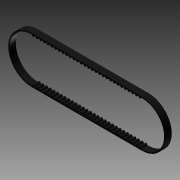
# Autodesk Inventor part: large drive belt
Saved by Autodesk Inventor 2012 (Build 160160000, 160)
## iProperties
Created: 2013-11-05
Part Number: large drive belt
Material: Default
Document SubType Name: Modeling
Designer: Bryce
Density: 1 g/cm^3
Author: Bryce
Autodesk Inventor part; units mm, degrees
ref_plane "YZ Plane" through (0, 0, 0) normal (1, 0, 0) x (0, 1, 0)
ref_plane "XZ Plane" through (0, 0, 0) normal (0, 1, 0) x (-1, 0, 0)
ref_plane "XY Plane" through (0, 0, 0) normal (0, 0, 1) x (1, 0, 0)
sketch "Sketch1" plane through (0, 0, 0) normal (0, 0, 1) x (1, 0, 0)
  arc A0 (0, 31.2674) -> (0, -31.2674) centre (0, 0) ccw
  arc A1 (155.575, -31.2674) -> (155.575, 31.2674) centre (155.575, 0) ccw
  line L0 (0, 31.2674) -> (155.575, 31.2674)
  line L1 (0, -31.2674) -> (4.3647, -31.2674)
  arc A2 (155.575, -33.02) -> (155.575, 33.02) centre (155.575, 0) ccw
  line L2 (155.575, -33.02) -> (0, -33.02)
  arc A3 (0, 33.02) -> (0, -33.02) centre (0, 0) ccw
  line L3 (0, 33.02) -> (155.575, 33.02)
  arc A4 (3.7592, -30.7283) -> (0.6055, -30.7283) centre (2.1824, -30.9118) ccw
  arc A5 (0, -31.2674) -> (0.6055, -30.7283) centre (0, -30.6578) ccw
  arc A6 (3.7592, -30.7283) -> (4.3647, -31.2674) centre (4.3647, -30.6578) ccw
  line L4 (4.3647, -31.2674) -> (155.575, -31.2674)
  line L5 (5.1816, -31.2674) -> (9.5463, -31.2674)
  arc A7 (8.9408, -30.7283) -> (5.7871, -30.7283) centre (7.364, -30.9118) ccw
  arc A8 (5.1816, -31.2674) -> (5.7871, -30.7283) centre (5.1816, -30.6578) ccw
  arc A9 (8.9408, -30.7283) -> (9.5463, -31.2674) centre (9.5463, -30.6578) ccw
  line L6 (10.3632, -31.2674) -> (14.7279, -31.2674)
  arc A10 (14.1224, -30.7283) -> (10.9687, -30.7283) centre (12.5456, -30.9118) ccw
  arc A11 (10.3632, -31.2674) -> (10.9687, -30.7283) centre (10.3632, -30.6578) ccw
  arc A12 (14.1224, -30.7283) -> (14.7279, -31.2674) centre (14.7279, -30.6578) ccw
  line L7 (15.5448, -31.2674) -> (19.9095, -31.2674)
  arc A13 (19.304, -30.7283) -> (16.1503, -30.7283) centre (17.7272, -30.9118) ccw
  arc A14 (15.5448, -31.2674) -> (16.1503, -30.7283) centre (15.5448, -30.6578) ccw
  arc A15 (19.304, -30.7283) -> (19.9095, -31.2674) centre (19.9095, -30.6578) ccw
  line L8 (20.7264, -31.2674) -> (25.0911, -31.2674)
  arc A16 (24.4856, -30.7283) -> (21.3319, -30.7283) centre (22.9088, -30.9118) ccw
  arc A17 (20.7264, -31.2674) -> (21.3319, -30.7283) centre (20.7264, -30.6578) ccw
  arc A18 (24.4856, -30.7283) -> (25.0911, -31.2674) centre (25.0911, -30.6578) ccw
  line L9 (25.908, -31.2674) -> (30.2727, -31.2674)
  arc A19 (29.6672, -30.7283) -> (26.5135, -30.7283) centre (28.0904, -30.9118) ccw
  arc A20 (25.908, -31.2674) -> (26.5135, -30.7283) centre (25.908, -30.6578) ccw
  arc A21 (29.6672, -30.7283) -> (30.2727, -31.2674) centre (30.2727, -30.6578) ccw
  line L10 (31.0896, -31.2674) -> (35.4543, -31.2674)
  arc A22 (34.8488, -30.7283) -> (31.6951, -30.7283) centre (33.272, -30.9118) ccw
  arc A23 (31.0896, -31.2674) -> (31.6951, -30.7283) centre (31.0896, -30.6578) ccw
  arc A24 (34.8488, -30.7283) -> (35.4543, -31.2674) centre (35.4543, -30.6578) ccw
  line L11 (36.2712, -31.2674) -> (40.6359, -31.2674)
  arc A25 (40.0304, -30.7283) -> (36.8767, -30.7283) centre (38.4536, -30.9118) ccw
  arc A26 (36.2712, -31.2674) -> (36.8767, -30.7283) centre (36.2712, -30.6578) ccw
  arc A27 (40.0304, -30.7283) -> (40.6359, -31.2674) centre (40.6359, -30.6578) ccw
  line L12 (41.4528, -31.2674) -> (45.8175, -31.2674)
  arc A28 (45.212, -30.7283) -> (42.0583, -30.7283) centre (43.6352, -30.9118) ccw
  arc A29 (41.4528, -31.2674) -> (42.0583, -30.7283) centre (41.4528, -30.6578) ccw
  arc A30 (45.212, -30.7283) -> (45.8175, -31.2674) centre (45.8175, -30.6578) ccw
  line L13 (46.6344, -31.2674) -> (50.9991, -31.2674)
  arc A31 (50.3936, -30.7283) -> (47.2399, -30.7283) centre (48.8168, -30.9118) ccw
  arc A32 (46.6344, -31.2674) -> (47.2399, -30.7283) centre (46.6344, -30.6578) ccw
  arc A33 (50.3936, -30.7283) -> (50.9991, -31.2674) centre (50.9991, -30.6578) ccw
  line L14 (51.816, -31.2674) -> (56.1807, -31.2674)
  arc A34 (55.5752, -30.7283) -> (52.4215, -30.7283) centre (53.9984, -30.9118) ccw
  arc A35 (51.816, -31.2674) -> (52.4215, -30.7283) centre (51.816, -30.6578) ccw
  arc A36 (55.5752, -30.7283) -> (56.1807, -31.2674) centre (56.1807, -30.6578) ccw
  line L15 (56.9976, -31.2674) -> (61.3623, -31.2674)
  arc A37 (60.7568, -30.7283) -> (57.6031, -30.7283) centre (59.18, -30.9118) ccw
  arc A38 (56.9976, -31.2674) -> (57.6031, -30.7283) centre (56.9976, -30.6578) ccw
  arc A39 (60.7568, -30.7283) -> (61.3623, -31.2674) centre (61.3623, -30.6578) ccw
  line L16 (62.1792, -31.2674) -> (66.5439, -31.2674)
  arc A40 (65.9384, -30.7283) -> (62.7847, -30.7283) centre (64.3616, -30.9118) ccw
  arc A41 (62.1792, -31.2674) -> (62.7847, -30.7283) centre (62.1792, -30.6578) ccw
  arc A42 (65.9384, -30.7283) -> (66.5439, -31.2674) centre (66.5439, -30.6578) ccw
  line L17 (67.3608, -31.2674) -> (71.7255, -31.2674)
  arc A43 (71.12, -30.7283) -> (67.9663, -30.7283) centre (69.5432, -30.9118) ccw
  arc A44 (67.3608, -31.2674) -> (67.9663, -30.7283) centre (67.3608, -30.6578) ccw
  arc A45 (71.12, -30.7283) -> (71.7255, -31.2674) centre (71.7255, -30.6578) ccw
  line L18 (72.5424, -31.2674) -> (76.9071, -31.2674)
  arc A46 (76.3016, -30.7283) -> (73.1479, -30.7283) centre (74.7248, -30.9118) ccw
  arc A47 (72.5424, -31.2674) -> (73.1479, -30.7283) centre (72.5424, -30.6578) ccw
  arc A48 (76.3016, -30.7283) -> (76.9071, -31.2674) centre (76.9071, -30.6578) ccw
  line L19 (77.724, -31.2674) -> (82.0887, -31.2674)
  arc A49 (81.4832, -30.7283) -> (78.3295, -30.7283) centre (79.9064, -30.9118) ccw
  arc A50 (77.724, -31.2674) -> (78.3295, -30.7283) centre (77.724, -30.6578) ccw
  arc A51 (81.4832, -30.7283) -> (82.0887, -31.2674) centre (82.0887, -30.6578) ccw
  line L20 (82.9056, -31.2674) -> (87.2703, -31.2674)
  arc A52 (86.6648, -30.7283) -> (83.5111, -30.7283) centre (85.088, -30.9118) ccw
  arc A53 (82.9056, -31.2674) -> (83.5111, -30.7283) centre (82.9056, -30.6578) ccw
  arc A54 (86.6648, -30.7283) -> (87.2703, -31.2674) centre (87.2703, -30.6578) ccw
  line L21 (88.0872, -31.2674) -> (92.4519, -31.2674)
  arc A55 (91.8464, -30.7283) -> (88.6927, -30.7283) centre (90.2696, -30.9118) ccw
  arc A56 (88.0872, -31.2674) -> (88.6927, -30.7283) centre (88.0872, -30.6578) ccw
  arc A57 (91.8464, -30.7283) -> (92.4519, -31.2674) centre (92.4519, -30.6578) ccw
  line L22 (93.2688, -31.2674) -> (97.6335, -31.2674)
  arc A58 (97.028, -30.7283) -> (93.8743, -30.7283) centre (95.4512, -30.9118) ccw
  arc A59 (93.2688, -31.2674) -> (93.8743, -30.7283) centre (93.2688, -30.6578) ccw
  arc A60 (97.028, -30.7283) -> (97.6335, -31.2674) centre (97.6335, -30.6578) ccw
  line L23 (98.4504, -31.2674) -> (102.8151, -31.2674)
  arc A61 (102.2096, -30.7283) -> (99.0559, -30.7283) centre (100.6328, -30.9118) ccw
  arc A62 (98.4504, -31.2674) -> (99.0559, -30.7283) centre (98.4504, -30.6578) ccw
  arc A63 (102.2096, -30.7283) -> (102.8151, -31.2674) centre (102.8151, -30.6578) ccw
  line L24 (103.632, -31.2674) -> (107.9967, -31.2674)
  arc A64 (107.3912, -30.7283) -> (104.2375, -30.7283) centre (105.8144, -30.9118) ccw
  arc A65 (103.632, -31.2674) -> (104.2375, -30.7283) centre (103.632, -30.6578) ccw
  arc A66 (107.3912, -30.7283) -> (107.9967, -31.2674) centre (107.9967, -30.6578) ccw
  line L25 (108.8136, -31.2674) -> (113.1783, -31.2674)
  arc A67 (112.5728, -30.7283) -> (109.4191, -30.7283) centre (110.996, -30.9118) ccw
  arc A68 (108.8136, -31.2674) -> (109.4191, -30.7283) centre (108.8136, -30.6578) ccw
  arc A69 (112.5728, -30.7283) -> (113.1783, -31.2674) centre (113.1783, -30.6578) ccw
  line L26 (113.9952, -31.2674) -> (118.3599, -31.2674)
  arc A70 (117.7544, -30.7283) -> (114.6007, -30.7283) centre (116.1776, -30.9118) ccw
  arc A71 (113.9952, -31.2674) -> (114.6007, -30.7283) centre (113.9952, -30.6578) ccw
  arc A72 (117.7544, -30.7283) -> (118.3599, -31.2674) centre (118.3599, -30.6578) ccw
  line L27 (119.1768, -31.2674) -> (123.5415, -31.2674)
  arc A73 (122.936, -30.7283) -> (119.7823, -30.7283) centre (121.3592, -30.9118) ccw
  arc A74 (119.1768, -31.2674) -> (119.7823, -30.7283) centre (119.1768, -30.6578) ccw
  arc A75 (122.936, -30.7283) -> (123.5415, -31.2674) centre (123.5415, -30.6578) ccw
  line L28 (124.3584, -31.2674) -> (128.7231, -31.2674)
  arc A76 (128.1176, -30.7283) -> (124.9639, -30.7283) centre (126.5408, -30.9118) ccw
  arc A77 (124.3584, -31.2674) -> (124.9639, -30.7283) centre (124.3584, -30.6578) ccw
  arc A78 (128.1176, -30.7283) -> (128.7231, -31.2674) centre (128.7231, -30.6578) ccw
  line L29 (129.54, -31.2674) -> (133.9047, -31.2674)
  arc A79 (133.2992, -30.7283) -> (130.1455, -30.7283) centre (131.7224, -30.9118) ccw
  arc A80 (129.54, -31.2674) -> (130.1455, -30.7283) centre (129.54, -30.6578) ccw
  arc A81 (133.2992, -30.7283) -> (133.9047, -31.2674) centre (133.9047, -30.6578) ccw
  line L30 (134.7216, -31.2674) -> (139.0863, -31.2674)
  arc A82 (138.4808, -30.7283) -> (135.3271, -30.7283) centre (136.904, -30.9118) ccw
  arc A83 (134.7216, -31.2674) -> (135.3271, -30.7283) centre (134.7216, -30.6578) ccw
  arc A84 (138.4808, -30.7283) -> (139.0863, -31.2674) centre (139.0863, -30.6578) ccw
  line L31 (139.9032, -31.2674) -> (144.2679, -31.2674)
  arc A85 (143.6624, -30.7283) -> (140.5087, -30.7283) centre (142.0856, -30.9118) ccw
  arc A86 (139.9032, -31.2674) -> (140.5087, -30.7283) centre (139.9032, -30.6578) ccw
  arc A87 (143.6624, -30.7283) -> (144.2679, -31.2674) centre (144.2679, -30.6578) ccw
  line L32 (145.0848, -31.2674) -> (149.4495, -31.2674)
  arc A88 (148.844, -30.7283) -> (145.6903, -30.7283) centre (147.2672, -30.9118) ccw
  arc A89 (145.0848, -31.2674) -> (145.6903, -30.7283) centre (145.0848, -30.6578) ccw
  arc A90 (148.844, -30.7283) -> (149.4495, -31.2674) centre (149.4495, -30.6578) ccw
  line L33 (150.2664, -31.2674) -> (154.6311, -31.2674)
  arc A91 (154.0256, -30.7283) -> (150.8719, -30.7283) centre (152.4488, -30.9118) ccw
  arc A92 (150.2664, -31.2674) -> (150.8719, -30.7283) centre (150.2664, -30.6578) ccw
  arc A93 (154.0256, -30.7283) -> (154.6311, -31.2674) centre (154.6311, -30.6578) ccw
  line L34 (0, 0) -> (155.575, 0) construction
  line L35 (0, 31.2674) -> (4.3647, 31.2674)
  arc A94 (0.6055, 30.7283) -> (3.7592, 30.7283) centre (2.1824, 30.9118) ccw
  arc A95 (0.6055, 30.7283) -> (0, 31.2674) centre (0, 30.6578) ccw
  arc A96 (4.3647, 31.2674) -> (3.7592, 30.7283) centre (4.3647, 30.6578) ccw
  line L36 (5.1816, 31.2674) -> (9.5463, 31.2674)
  arc A97 (5.7871, 30.7283) -> (8.9408, 30.7283) centre (7.364, 30.9118) ccw
  arc A98 (5.7871, 30.7283) -> (5.1816, 31.2674) centre (5.1816, 30.6578) ccw
  arc A99 (9.5463, 31.2674) -> (8.9408, 30.7283) centre (9.5463, 30.6578) ccw
  line L37 (10.3632, 31.2674) -> (14.7279, 31.2674)
  arc A100 (10.9687, 30.7283) -> (14.1224, 30.7283) centre (12.5456, 30.9118) ccw
  arc A101 (10.9687, 30.7283) -> (10.3632, 31.2674) centre (10.3632, 30.6578) ccw
  arc A102 (14.7279, 31.2674) -> (14.1224, 30.7283) centre (14.7279, 30.6578) ccw
  line L38 (15.5448, 31.2674) -> (19.9095, 31.2674)
  arc A103 (16.1503, 30.7283) -> (19.304, 30.7283) centre (17.7272, 30.9118) ccw
  arc A104 (16.1503, 30.7283) -> (15.5448, 31.2674) centre (15.5448, 30.6578) ccw
  arc A105 (19.9095, 31.2674) -> (19.304, 30.7283) centre (19.9095, 30.6578) ccw
  line L39 (20.7264, 31.2674) -> (25.0911, 31.2674)
  arc A106 (21.3319, 30.7283) -> (24.4856, 30.7283) centre (22.9088, 30.9118) ccw
  arc A107 (21.3319, 30.7283) -> (20.7264, 31.2674) centre (20.7264, 30.6578) ccw
  arc A108 (25.0911, 31.2674) -> (24.4856, 30.7283) centre (25.0911, 30.6578) ccw
  line L40 (25.908, 31.2674) -> (30.2727, 31.2674)
  arc A109 (26.5135, 30.7283) -> (29.6672, 30.7283) centre (28.0904, 30.9118) ccw
  arc A110 (26.5135, 30.7283) -> (25.908, 31.2674) centre (25.908, 30.6578) ccw
  arc A111 (30.2727, 31.2674) -> (29.6672, 30.7283) centre (30.2727, 30.6578) ccw
  line L41 (31.0896, 31.2674) -> (35.4543, 31.2674)
  arc A112 (31.6951, 30.7283) -> (34.8488, 30.7283) centre (33.272, 30.9118) ccw
  arc A113 (31.6951, 30.7283) -> (31.0896, 31.2674) centre (31.0896, 30.6578) ccw
  arc A114 (35.4543, 31.2674) -> (34.8488, 30.7283) centre (35.4543, 30.6578) ccw
  line L42 (36.2712, 31.2674) -> (40.6359, 31.2674)
  arc A115 (36.8767, 30.7283) -> (40.0304, 30.7283) centre (38.4536, 30.9118) ccw
  arc A116 (36.8767, 30.7283) -> (36.2712, 31.2674) centre (36.2712, 30.6578) ccw
  arc A117 (40.6359, 31.2674) -> (40.0304, 30.7283) centre (40.6359, 30.6578) ccw
  line L43 (41.4528, 31.2674) -> (45.8175, 31.2674)
  arc A118 (42.0583, 30.7283) -> (45.212, 30.7283) centre (43.6352, 30.9118) ccw
  arc A119 (42.0583, 30.7283) -> (41.4528, 31.2674) centre (41.4528, 30.6578) ccw
  arc A120 (45.8175, 31.2674) -> (45.212, 30.7283) centre (45.8175, 30.6578) ccw
  line L44 (46.6344, 31.2674) -> (50.9991, 31.2674)
  arc A121 (47.2399, 30.7283) -> (50.3936, 30.7283) centre (48.8168, 30.9118) ccw
  arc A122 (47.2399, 30.7283) -> (46.6344, 31.2674) centre (46.6344, 30.6578) ccw
  arc A123 (50.9991, 31.2674) -> (50.3936, 30.7283) centre (50.9991, 30.6578) ccw
  line L45 (51.816, 31.2674) -> (56.1807, 31.2674)
  arc A124 (52.4215, 30.7283) -> (55.5752, 30.7283) centre (53.9984, 30.9118) ccw
  arc A125 (52.4215, 30.7283) -> (51.816, 31.2674) centre (51.816, 30.6578) ccw
  arc A126 (56.1807, 31.2674) -> (55.5752, 30.7283) centre (56.1807, 30.6578) ccw
  line L46 (56.9976, 31.2674) -> (61.3623, 31.2674)
  arc A127 (57.6031, 30.7283) -> (60.7568, 30.7283) centre (59.18, 30.9118) ccw
  arc A128 (57.6031, 30.7283) -> (56.9976, 31.2674) centre (56.9976, 30.6578) ccw
  arc A129 (61.3623, 31.2674) -> (60.7568, 30.7283) centre (61.3623, 30.6578) ccw
  line L47 (62.1792, 31.2674) -> (66.5439, 31.2674)
  arc A130 (62.7847, 30.7283) -> (65.9384, 30.7283) centre (64.3616, 30.9118) ccw
  arc A131 (62.7847, 30.7283) -> (62.1792, 31.2674) centre (62.1792, 30.6578) ccw
  arc A132 (66.5439, 31.2674) -> (65.9384, 30.7283) centre (66.5439, 30.6578) ccw
  line L48 (67.3608, 31.2674) -> (71.7255, 31.2674)
  arc A133 (67.9663, 30.7283) -> (71.12, 30.7283) centre (69.5432, 30.9118) ccw
  arc A134 (67.9663, 30.7283) -> (67.3608, 31.2674) centre (67.3608, 30.6578) ccw
  arc A135 (71.7255, 31.2674) -> (71.12, 30.7283) centre (71.7255, 30.6578) ccw
  line L49 (72.5424, 31.2674) -> (76.9071, 31.2674)
  arc A136 (73.1479, 30.7283) -> (76.3016, 30.7283) centre (74.7248, 30.9118) ccw
  arc A137 (73.1479, 30.7283) -> (72.5424, 31.2674) centre (72.5424, 30.6578) ccw
  arc A138 (76.9071, 31.2674) -> (76.3016, 30.7283) centre (76.9071, 30.6578) ccw
  line L50 (77.724, 31.2674) -> (82.0887, 31.2674)
  arc A139 (78.3295, 30.7283) -> (81.4832, 30.7283) centre (79.9064, 30.9118) ccw
  arc A140 (78.3295, 30.7283) -> (77.724, 31.2674) centre (77.724, 30.6578) ccw
  arc A141 (82.0887, 31.2674) -> (81.4832, 30.7283) centre (82.0887, 30.6578) ccw
  line L51 (82.9056, 31.2674) -> (87.2703, 31.2674)
  arc A142 (83.5111, 30.7283) -> (86.6648, 30.7283) centre (85.088, 30.9118) ccw
  arc A143 (83.5111, 30.7283) -> (82.9056, 31.2674) centre (82.9056, 30.6578) ccw
  arc A144 (87.2703, 31.2674) -> (86.6648, 30.7283) centre (87.2703, 30.6578) ccw
  line L52 (88.0872, 31.2674) -> (92.4519, 31.2674)
  arc A145 (88.6927, 30.7283) -> (91.8464, 30.7283) centre (90.2696, 30.9118) ccw
  arc A146 (88.6927, 30.7283) -> (88.0872, 31.2674) centre (88.0872, 30.6578) ccw
  arc A147 (92.4519, 31.2674) -> (91.8464, 30.7283) centre (92.4519, 30.6578) ccw
  line L53 (93.2688, 31.2674) -> (97.6335, 31.2674)
  arc A148 (93.8743, 30.7283) -> (97.028, 30.7283) centre (95.4512, 30.9118) ccw
  arc A149 (93.8743, 30.7283) -> (93.2688, 31.2674) centre (93.2688, 30.6578) ccw
  arc A150 (97.6335, 31.2674) -> (97.028, 30.7283) centre (97.6335, 30.6578) ccw
  line L54 (98.4504, 31.2674) -> (102.8151, 31.2674)
  arc A151 (99.0559, 30.7283) -> (102.2096, 30.7283) centre (100.6328, 30.9118) ccw
  arc A152 (99.0559, 30.7283) -> (98.4504, 31.2674) centre (98.4504, 30.6578) ccw
  arc A153 (102.8151, 31.2674) -> (102.2096, 30.7283) centre (102.8151, 30.6578) ccw
  line L55 (103.632, 31.2674) -> (107.9967, 31.2674)
  arc A154 (104.2375, 30.7283) -> (107.3912, 30.7283) centre (105.8144, 30.9118) ccw
  arc A155 (104.2375, 30.7283) -> (103.632, 31.2674) centre (103.632, 30.6578) ccw
  arc A156 (107.9967, 31.2674) -> (107.3912, 30.7283) centre (107.9967, 30.6578) ccw
  line L56 (108.8136, 31.2674) -> (113.1783, 31.2674)
  arc A157 (109.4191, 30.7283) -> (112.5728, 30.7283) centre (110.996, 30.9118) ccw
  arc A158 (109.4191, 30.7283) -> (108.8136, 31.2674) centre (108.8136, 30.6578) ccw
  arc A159 (113.1783, 31.2674) -> (112.5728, 30.7283) centre (113.1783, 30.6578) ccw
  line L57 (113.9952, 31.2674) -> (118.3599, 31.2674)
  arc A160 (114.6007, 30.7283) -> (117.7544, 30.7283) centre (116.1776, 30.9118) ccw
  arc A161 (114.6007, 30.7283) -> (113.9952, 31.2674) centre (113.9952, 30.6578) ccw
  arc A162 (118.3599, 31.2674) -> (117.7544, 30.7283) centre (118.3599, 30.6578) ccw
  line L58 (119.1768, 31.2674) -> (123.5415, 31.2674)
  arc A163 (119.7823, 30.7283) -> (122.936, 30.7283) centre (121.3592, 30.9118) ccw
  arc A164 (119.7823, 30.7283) -> (119.1768, 31.2674) centre (119.1768, 30.6578) ccw
  arc A165 (123.5415, 31.2674) -> (122.936, 30.7283) centre (123.5415, 30.6578) ccw
  line L59 (124.3584, 31.2674) -> (128.7231, 31.2674)
  arc A166 (124.9639, 30.7283) -> (128.1176, 30.7283) centre (126.5408, 30.9118) ccw
  arc A167 (124.9639, 30.7283) -> (124.3584, 31.2674) centre (124.3584, 30.6578) ccw
  arc A168 (128.7231, 31.2674) -> (128.1176, 30.7283) centre (128.7231, 30.6578) ccw
  line L60 (129.54, 31.2674) -> (133.9047, 31.2674)
  arc A169 (130.1455, 30.7283) -> (133.2992, 30.7283) centre (131.7224, 30.9118) ccw
  arc A170 (130.1455, 30.7283) -> (129.54, 31.2674) centre (129.54, 30.6578) ccw
  arc A171 (133.9047, 31.2674) -> (133.2992, 30.7283) centre (133.9047, 30.6578) ccw
  line L61 (134.7216, 31.2674) -> (139.0863, 31.2674)
  arc A172 (135.3271, 30.7283) -> (138.4808, 30.7283) centre (136.904, 30.9118) ccw
  arc A173 (135.3271, 30.7283) -> (134.7216, 31.2674) centre (134.7216, 30.6578) ccw
  arc A174 (139.0863, 31.2674) -> (138.4808, 30.7283) centre (139.0863, 30.6578) ccw
  line L62 (139.9032, 31.2674) -> (144.2679, 31.2674)
  arc A175 (140.5087, 30.7283) -> (143.6624, 30.7283) centre (142.0856, 30.9118) ccw
  arc A176 (140.5087, 30.7283) -> (139.9032, 31.2674) centre (139.9032, 30.6578) ccw
  arc A177 (144.2679, 31.2674) -> (143.6624, 30.7283) centre (144.2679, 30.6578) ccw
  line L63 (145.0848, 31.2674) -> (149.4495, 31.2674)
  arc A178 (145.6903, 30.7283) -> (148.844, 30.7283) centre (147.2672, 30.9118) ccw
  arc A179 (145.6903, 30.7283) -> (145.0848, 31.2674) centre (145.0848, 30.6578) ccw
  arc A180 (149.4495, 31.2674) -> (148.844, 30.7283) centre (149.4495, 30.6578) ccw
  line L64 (150.2664, 31.2674) -> (154.6311, 31.2674)
  arc A181 (150.8719, 30.7283) -> (154.0256, 30.7283) centre (152.4488, 30.9118) ccw
  arc A182 (150.8719, 30.7283) -> (150.2664, 31.2674) centre (150.2664, 30.6578) ccw
  arc A183 (154.6311, 31.2674) -> (154.0256, 30.7283) centre (154.6311, 30.6578) ccw
  dimension "d0" = 155.575
  dimension "d1" = 31.2674
  dimension "d2" = 33.02
  dimension "d4" = 1.5875
  dimension "d5" = 0.6096
  dimension "d6" = 0.254
  dimension "d9" = 5.1816
  dimension "d16" = 31.2674
  constraints: 368 point on circle, 209 symmetric about line, 184 centre point, 130 end point, 15 tangent, 1 coincident, 1 equal radius, 1 horizontal, 1 horizontal alignment, 410 other
  measures "d0" distance of L34.end point (0, 0)
  measures "d1" radius of A0
  measures "d2" radius of A3
  measures "d4" radius of A4
  measures "d5" radius of A5
  measures "d6" vertical distance of A4.centre A5.centre
  measures "d9" distance of L1.start L5.start
  measures "d16" radius of A1
extrude "Extrusion1" add sketch "Sketch1" along normal blind 9 contours L0 A96 A94 A95 | A5 A4 A6 L1 | L0 A99 A97 A98 | A8 A7 A9 L4 | L0 A102 A100 A101 | A11 A10 A12 L4 | L0 A105 A103 A104 | A14 A13 A15 L4 | L0 A108 A106 A107 | A17 A16 A18 L4 | L0 A111 A109 A110 | A20 A19 A21 L4 | L0 A114 A112 A113 | A23 A22 A24 L4 | L0 A117 A115 A116 | A26 A25 A27 L4 | L0 A120 A118 A119 | A29 A28 A30 L4 | L0 A123 A121 A122 | A32 A31 A33 L4 | L0 A126 A124 A125 | A35 A34 A36 L4 | L0 A129 A127 A128 | A38 A37 A39 L4 | L0 A132 A130 A131 | A41 A40 A42 L4 | L0 A135 A133 A134 | A44 A43 A45 L4 | L0 A138 A136 A137 | A47 A46 A48 L4 | L0 A141 A139 A140 | A50 A49 A51 L4 | L0 A144 A142 A143 | A53 A52 A54 L4 | L0 A147 A145 A146 | A56 A55 A57 L4 | L0 A150 A148 A149 | A59 A58 A60 L4 | L0 A153 A151 A152 | A62 A61 A63 L4 | L0 A156 A154 A155 | A65 A64 A66 L4 | L0 A159 A157 A158 | A68 A67 A69 L4 | L0 A162 A160 A161 | A71 A70 A72 L4 | L0 A165 A163 A164 | A74 A73 A75 L4 | L0 A168 A166 A167 | A77 A76 A78 L4 | L0 A171 A169 A170 | A80 A79 A81 L4 | L0 A174 A172 A173 | A83 A82 A84 L4 | L0 A177 A175 A176 | A86 A85 A87 L4 | L0 A180 A178 A179 | A89 A88 A90 L4 | L0 A183 A181 A182 | A92 A91 A93 L4 | L2 A3 L3 A2
body "Solid1"
